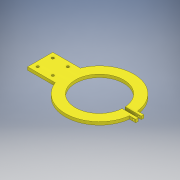
# Autodesk Inventor part: motor_hold_sample
Saved by Autodesk Inventor 2018 (Build 220112000, 112)
## iProperties
Created: 2017-10-24
Part Number: motor_hold_sample
Material: アルミニウム 6061
Document SubType Name: Modeling
Designer: 翔
Density: 2.7 g/cm^3
Appearance: カナリア
Author: 翔
Autodesk Inventor part; units mm, degrees
ref_plane "YZ Plane" through (0, 0, 0) normal (1, 0, 0) x (0, 1, 0)
ref_plane "XZ Plane" through (0, 0, 0) normal (0, 1, 0) x (-1, 0, 0)
ref_plane "XY Plane" through (0, 0, 0) normal (0, 0, 1) x (1, 0, 0)
sketch "スケッチ2" plane through (0, 0, 0) normal (0, 0, 1) x (1, 0, 0)
  line L0 (0, -106.3056) -> (0, 106.3056) projected
  line L1 (-64.6, 0) -> (212.6, 0) projected
  arc A0 (140.9062, 3) -> (140.9062, -3) centre (93, 0) ccw
  line L2 (-25, -25) -> (25, -25)
  line L3 (25, 25) -> (-25, 25)
  line L4 (-25, -25) -> (25, 25) construction
  line L5 (25, -25) -> (-25, 25) construction
  line L6 (25, 25) -> (29.7624, 25)
  line L7 (25, -25) -> (29.7624, -25)
  line L8 (140.9062, -3) -> (173, -3)
  line L9 (173, 3) -> (140.9062, 3)
  line L10 (145.3369, -0.7898) -> (173, 3) construction
  line L11 (173, -3) -> (145.3176, 0.7925) construction
  arc A1 (29.7624, -25) -> (160.5278, -8) centre (93, 0) ccw
  arc A2 (160.5278, 8) -> (29.7624, 25) centre (93, 0) ccw
  line L12 (173, 3) -> (173, 8)
  line L13 (173, 8) -> (160.5278, 8)
  line L14 (173, -3) -> (173, -8)
  line L15 (173, -8) -> (160.5278, -8)
  line L16 (-25, 25) -> (-25, -25)
  point P0 (0, 0)
  point P1 (151.102, 0)
  dimension "d1" = 96
  dimension "d2" = 50
  dimension "d7" = 5
  dimension "d8" = 3
  dimension "d9" = 5
  dimension "d10" = 80
  dimension "d12" = 20
  dimension "d13" = 93
  dimension "d15" = 20
  dimension "d16" = 50
  dimension "d17" = 3
  dimension "d18" = 50
  constraints: 30 end point, 6 point on circle, 5 point on line, 3 centre point, 3 horizontal, 3 parallel, 3 perpendicular, 2 midpoint, 1 vertical
  measures "d1" diameter of A0
  measures "d2" distance of L3.start L3.end
  measures "d7" distance between parallel lines of L9 L13
  measures "d8" distance from line of point (151.102, 0) L9
  measures "d9" distance between parallel lines of L15 L8
  measures "d10" distance from line of A0.centre L14
  measures "d12" radial gap between concentric circles of A2 A0
  measures "d13" distance of point (0, 0) A0.centre
  measures "d15" radial gap between concentric circles of A1 A0
  measures "d16" distance of L2.start L2.end
  measures "d17" distance from line of point (151.102, 0) L8
  measures "d18" distance of L3.end L2.start
extrude "押し出し1" add sketch "スケッチ2" along normal blind 6
sketch "スケッチ3" plane through (0, 0, 6) normal (0, 0, 1) x (1, 0, 0)
  line L0 (15, -15) -> (-15, -15)
  line L1 (-15, -15) -> (-15, 15)
  line L2 (-15, 15) -> (15, 15)
  line L3 (15, 15) -> (15, -15)
  line L4 (15, -15) -> (-15, 15) construction
  line L5 (-15, -15) -> (15, 15) construction
  circle A0 centre (-15, -15) radius 2.5
  circle A1 centre (-15, 15) radius 2.5
  line L6 (-15, 15) -> (-15, 45)
  circle A2 centre (15, -15) radius 2.5
  circle A3 centre (15, 15) radius 2.5
  point P0 (0, 0)
  dimension "d21" = 30
  dimension "d22" = 30
  dimension "d23" = 5
  dimension "d26" = 30
  dimension "d33" = 30
  constraints: 14 end point, 4 centre point, 2 coincident, 2 horizontal, 2 midpoint, 2 parallel, 1 collinear, 1 perpendicular, 1 vertical, 8 other
  measures "d21" distance of L0.end L1.end
  measures "d22" distance of L1.end L2.end
  measures "d23" diameter of A0
  measures "d26" distance of A0.centre A1.centre
  measures "d33" distance of A0.centre A2.centre
extrude "押し出し2" cut sketch "スケッチ3" against normal blind 6 contours A0 L1 L0 | L0 L1 A0 | A2 L3 L0 | L0 L3 A2 | A1 L6 L1 | L1 L2 A1 | A3 L2 L3 | L3 L2 A3 | L6 A1 L2
sketch "スケッチ4" plane through (160.5278, -8, 0) normal (0, -1, 0) x (1, 0, 0)
  circle A0 centre (7.4722, 3) radius 2
  line L0 (0, 0) -> (12.4722, 0) projected
  line L1 (12.4722, 0) -> (12.4722, 6) projected
  point P0 (-160.5278, 0)
  dimension "d40" = 3
  dimension "d41" = 4
  dimension "d42" = 5
  constraints: 1 centre point
  measures "d40" distance from line of A0.centre L0
  measures "d41" diameter of A0
  measures "d42" distance from line of L1 A0.centre
extrude "押し出し3" cut sketch "スケッチ4" against normal through all
